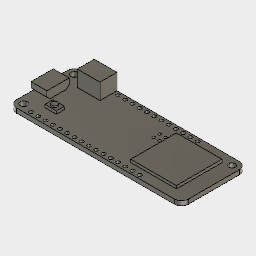
3027 Adafruit FONA Feather 32u4 (Autodesk Fusion 360 design; units mm, degrees)
Autodesk Fusion 360 part; units mm, degrees
sketch "Adafruit Feather 32u4 FONA" plane through (0, 0, 0) normal (0, 0, 1) x (1, 0, 0)
  arc A0 (1.895, 14.93) -> (2.295, 14.58) centre (2.27, 14.955) ccw
  line L0 (0, 8.89) -> (0, 2.54)
  arc A1 (60.325, 20.32) -> (57.785, 22.86) centre (57.785, 20.32) ccw
  arc A2 (2.245, 8.28) -> (1.895, 7.83) centre (2.295, 7.88) ccw
  arc A3 (57.785, 0) -> (60.325, 2.54) centre (57.785, 2.54) ccw
  line L1 (2.845, 14.58) -> (2.295, 14.58)
  line L2 (1.895, 14.93) -> (1.895, 15.13)
  arc A4 (1.895, 7.83) -> (2.245, 7.38) centre (2.295, 7.78) ccw
  arc A5 (0, 2.54) -> (2.54, 0) centre (2.54, 2.54) ccw
  arc A6 (2.845, 14.58) -> (3.195, 14.93) centre (2.845, 14.93) ccw
  arc A7 (2.54, 22.86) -> (0, 20.32) centre (2.54, 20.32) ccw
  line L3 (57.785, 22.86) -> (2.54, 22.86)
  line L4 (60.325, 2.54) -> (60.325, 20.32)
  arc A8 (2.295, 15.48) -> (1.895, 15.13) centre (2.27, 15.105) ccw
  line L5 (3.195, 15.13) -> (3.195, 14.93)
  circle A9 centre (57.785, 20.32) radius 1.1
  line L6 (2.54, 0) -> (57.785, 0)
  arc A10 (3.195, 7.83) -> (2.845, 8.28) centre (2.795, 7.88) ccw
  line L7 (0.508, 13.589) -> (0.508, 9.398)
  line L8 (2.845, 7.38) -> (2.245, 7.38)
  line L9 (0.508, 9.398) -> (0, 8.89)
  line L10 (2.245, 8.28) -> (2.845, 8.28)
  line L11 (0, 20.32) -> (0, 14.097)
  line L12 (0, 14.097) -> (0.508, 13.589)
  arc A11 (2.845, 7.38) -> (3.195, 7.83) centre (2.795, 7.78) ccw
  circle A12 centre (4.445, 13.38) radius 0.35
  arc A13 (3.195, 15.13) -> (2.845, 15.48) centre (2.845, 15.13) ccw
  circle A14 centre (4.445, 9.48) radius 0.35
  line L13 (2.295, 15.48) -> (2.845, 15.48)
  circle A15 centre (35.576, 15.113) radius 0.704
  line L14 (3.795, 9.08) -> (1.295, 9.08)
  circle A16 centre (35.576, 17.145) radius 0.704
  circle A17 centre (39.37, 1.27) radius 0.8382
  line L15 (1.295, 9.08) -> (1.295, 6.58)
  line L16 (1.295, 16.28) -> (1.295, 13.78)
  arc A18 (5.999, 8.13) -> (4.691, 8.13) centre (5.345, 8.13) ccw
  circle A19 centre (35.576, 17.145) radius 0.704
  line L17 (3.795, 16.28) -> (1.295, 16.28)
  line L18 (3.795, 6.58) -> (3.795, 9.08)
  line L19 (1.295, 9.08) -> (1.295, 6.58)
  line L20 (5.999, 6.822) -> (5.999, 8.13)
  line L21 (1.295, 13.78) -> (3.795, 13.78)
  line L22 (4.691, 8.13) -> (4.691, 6.822)
  arc A20 (5.999, 8.13) -> (4.691, 8.13) centre (5.345, 8.13) ccw
  arc A21 (4.691, 6.822) -> (5.999, 6.822) centre (5.345, 6.822) ccw
  line L23 (5.999, 6.822) -> (5.999, 8.13)
  line L24 (3.795, 13.78) -> (3.795, 16.28)
  circle A22 centre (37.576, 17.145) radius 0.704
  line L25 (3.795, 9.08) -> (1.295, 9.08)
  circle A23 centre (37.576, 17.145) radius 0.704
  line L26 (1.295, 13.78) -> (3.795, 13.78)
  arc A24 (4.691, 6.822) -> (5.999, 6.822) centre (5.345, 6.822) ccw
  line L27 (1.295, 16.28) -> (1.295, 13.78)
  line L28 (1.295, 6.58) -> (3.795, 6.58)
  arc A25 (5.999, 16.038) -> (4.691, 16.038) centre (5.345, 16.038) ccw
  line L29 (3.795, 13.78) -> (3.795, 16.28)
  line L30 (5.999, 14.73) -> (5.999, 16.038)
  line L31 (5.999, 14.73) -> (5.999, 16.038)
  arc A26 (4.691, 14.73) -> (5.999, 14.73) centre (5.345, 14.73) ccw
  arc A27 (5.999, 16.038) -> (4.691, 16.038) centre (5.345, 16.038) ccw
  line L32 (4.691, 16.038) -> (4.691, 14.73)
  line L33 (4.691, 8.13) -> (4.691, 6.822)
  line L34 (3.795, 6.58) -> (3.795, 9.08)
  arc A28 (4.691, 14.73) -> (5.999, 14.73) centre (5.345, 14.73) ccw
  line L35 (1.295, 6.58) -> (3.795, 6.58)
  line L36 (4.691, 16.038) -> (4.691, 14.73)
  circle A29 centre (37.576, 15.113) radius 0.704
  circle A30 centre (37.576, 15.113) radius 0.704
  circle A31 centre (35.576, 15.113) radius 0.704
  line L37 (3.795, 16.28) -> (1.295, 16.28)
  circle A32 centre (21.59, 21.59) radius 0.8382
  circle A33 centre (41.91, 1.27) radius 0.8382
  circle A34 centre (44.45, 1.27) radius 0.8382
  circle A35 centre (41.91, 1.27) radius 0.8382
  circle A36 centre (2.54, 20.32) radius 1.758
  circle A37 centre (2.54, 2.54) radius 1.758
  circle A38 centre (2.54, 2.54) radius 1.758
  circle A39 centre (2.54, 20.32) radius 1.758
  circle A40 centre (24.13, 21.59) radius 0.8382
  circle A41 centre (21.59, 21.59) radius 0.8382
  circle A42 centre (24.13, 21.59) radius 0.8382
  circle A43 centre (41.91, 21.59) radius 0.8382
  circle A44 centre (41.91, 21.59) radius 0.8382
  circle A45 centre (44.45, 21.59) radius 0.8382
  circle A46 centre (44.45, 21.59) radius 0.8382
  circle A47 centre (36.83, 21.59) radius 0.8382
  circle A48 centre (19.05, 21.59) radius 0.8382
  circle A49 centre (16.51, 21.59) radius 0.8382
  circle A50 centre (21.59, 1.27) radius 0.8382
  circle A51 centre (21.59, 1.27) radius 0.8382
  circle A52 centre (24.13, 1.27) radius 0.8382
  circle A53 centre (11.43, 1.27) radius 0.8382
  circle A54 centre (19.05, 21.59) radius 0.8382
  circle A55 centre (24.13, 1.27) radius 0.8382
  circle A56 centre (26.67, 1.27) radius 0.8382
  circle A57 centre (16.51, 1.27) radius 0.8382
  circle A58 centre (16.51, 1.27) radius 0.8382
  circle A59 centre (16.51, 21.59) radius 0.8382
  circle A60 centre (39.37, 21.59) radius 0.8382
  circle A61 centre (36.83, 21.59) radius 0.8382
  circle A62 centre (39.37, 21.59) radius 0.8382
  circle A63 centre (31.75, 1.27) radius 0.8382
  circle A64 centre (31.75, 1.27) radius 0.8382
  circle A65 centre (29.21, 1.27) radius 0.8382
  circle A66 centre (29.21, 1.27) radius 0.8382
  circle A67 centre (26.67, 1.27) radius 0.8382
  circle A68 centre (8.89, 1.27) radius 0.8382
  circle A69 centre (34.29, 1.27) radius 0.8382
  circle A70 centre (6.35, 1.27) radius 0.8382
  circle A71 centre (8.89, 1.27) radius 0.8382
  circle A72 centre (6.35, 1.27) radius 0.8382
  circle A73 centre (31.75, 21.59) radius 0.8382
  circle A74 centre (31.75, 21.59) radius 0.8382
  circle A75 centre (34.29, 21.59) radius 0.8382
  circle A76 centre (34.29, 1.27) radius 0.8382
  circle A77 centre (29.21, 21.59) radius 0.8382
  circle A78 centre (34.29, 21.59) radius 0.8382
  circle A79 centre (26.67, 21.59) radius 0.8382
  circle A80 centre (11.43, 1.27) radius 0.8382
  circle A81 centre (39.37, 1.27) radius 0.8382
  circle A82 centre (13.97, 1.27) radius 0.8382
  circle A83 centre (26.67, 21.59) radius 0.8382
  circle A84 centre (36.83, 1.27) radius 0.8382
  circle A85 centre (44.45, 1.27) radius 0.8382
  circle A86 centre (19.05, 1.27) radius 0.8382
  circle A87 centre (19.05, 1.27) radius 0.8382
  circle A88 centre (13.97, 1.27) radius 0.8382
  circle A89 centre (29.21, 21.59) radius 0.8382
  circle A90 centre (36.83, 1.27) radius 0.8382
  circle A91 centre (2.54, 2.54) radius 1.25
  circle A92 centre (2.54, 20.32) radius 1.25
  dimension "d1" = 2.5
  dimension "d2" = 2.5
  measures "d1" diameter of A91
  measures "d2" diameter of A92
extrude "Extrude1" add sketch "Adafruit Feather 32u4 FONA" against normal blind 1.6 contours A0 L1 L2 A6 A8 L5 A13 L13 | L0 A1 A3 A5 A7 L3 L4 L6 L7 L9 L11 L12 | A2 A4 A10 L8 L10 A11 | A12 | A14 | L14 L15 L18 L19 L25 L28 L34 L35 | L16 L17 L21 L24 L26 L27 L29 L37 | A18 L20 L22 A20 A21 L23 A24 L33 | A25 L30 L31 A26 A27 L32 A28 L36 | A36 A39 | A37 A38 makes body 1
move_face "OffsetFaces1" offset 0.203 32 faces at (44.5542, 2.1017, -1.0667) (42.0142, 2.1017, -1.0667) (39.4742, 2.1017, -1.0667) (36.9342, 2.1017, -1.0667) (34.3942, 2.1017, -1.0667) (32.2048, 1.9741, -1.0667) (30.044, 1.1865, -1.0667) (27.504, 1.1865, -1.0667) (24.964, 1.1865, -1.0667) (22.424, 1.1865, -1.0667) (19.884, 1.1865, -1.0667) (17.344, 1.1865, -1.0667) (14.804, 1.1865, -1.0667) (12.264, 1.1865, -1.0667) (9.724, 1.1865, -1.0667) (7.184, 1.1865, -1.0667) (17.3316, 21.4239, -1.0667) (19.8716, 21.4239, -1.0667) (22.4116, 21.4239, -1.0667) (24.9516, 21.4239, -1.0667) (27.4916, 21.4239, -1.0667) (30.0316, 21.4239, -1.0667) (32.2048, 22.2941, -1.0667) (33.6218, 22.0961, -1.0667) (36.1618, 22.0961, -1.0667) (38.7018, 22.0961, -1.0667) (41.2418, 22.0961, -1.0667) (43.7818, 22.0961, -1.0667) (37.958, 15.7044, -1.0667) (35.958, 15.7044, -1.0667) (35.958, 17.7364, -1.0667) (37.958, 17.7364, -1.0667) on bodies 1
sketch "microUSB" plane through (0, 0, 0) normal (0, 0, 1) x (-1, 0, 0)
  circle A0 centre (-36.83, -21.59) radius 0.6352
  circle A1 centre (-44.45, -21.59) radius 0.6352
  circle A2 centre (-29.21, -1.27) radius 0.6352
  circle A3 centre (-26.67, -1.27) radius 0.6352
  circle A4 centre (-8.89, -1.27) radius 0.6352
  circle A5 centre (-35.576, -17.145) radius 0.501
  circle A6 centre (-36.83, -1.27) radius 0.6352
  circle A7 centre (-29.21, -21.59) radius 0.6352
  circle A8 centre (-13.97, -1.27) radius 0.6352
  circle A9 centre (-19.05, -1.27) radius 0.6352
  circle A10 centre (-44.45, -1.27) radius 0.6352
  circle A11 centre (-26.67, -21.59) radius 0.6352
  circle A12 centre (-39.37, -1.27) radius 0.6352
  circle A13 centre (-39.37, -21.59) radius 0.6352
  circle A14 centre (-41.91, -1.27) radius 0.6352
  circle A15 centre (-6.35, -1.27) radius 0.6352
  circle A16 centre (-16.51, -21.59) radius 0.6352
  circle A17 centre (-16.51, -1.27) radius 0.6352
  circle A18 centre (-19.05, -21.59) radius 0.6352
  circle A19 centre (-31.75, -1.27) radius 0.6352
  circle A20 centre (-21.59, -1.27) radius 0.6352
  circle A21 centre (-11.43, -1.27) radius 0.6352
  circle A22 centre (-37.576, -15.113) radius 0.501
  circle A23 centre (-57.785, -20.32) radius 1.1
  circle A24 centre (-2.54, -20.32) radius 1.25
  circle A25 centre (-2.54, -2.54) radius 1.25
  circle A26 centre (-37.576, -17.145) radius 0.501
  circle A27 centre (-35.576, -15.113) radius 0.501
  circle A28 centre (-31.75, -21.59) radius 0.6352
  circle A29 centre (-24.13, -1.27) radius 0.6352
  circle A30 centre (-34.29, -21.59) radius 0.6352
  circle A31 centre (-41.91, -21.59) radius 0.6352
  circle A32 centre (-21.59, -21.59) radius 0.6352
  circle A33 centre (-34.29, -1.27) radius 0.6352
  circle A34 centre (-24.13, -21.59) radius 0.6352
  line L0 (0, -14.097) -> (-0.508, -13.589)
  line L1 (-0.508, -13.589) -> (-0.508, -9.398)
  line L2 (-0.508, -9.398) -> (0, -8.89)
  line L3 (0, -8.89) -> (0, -2.54)
  arc A35 (0, -2.54) -> (-2.54, 0) centre (-2.54, -2.54) ccw
  line L4 (-2.54, 0) -> (-57.785, 0)
  arc A36 (-57.785, 0) -> (-60.325, -2.54) centre (-57.785, -2.54) ccw
  line L5 (-60.325, -2.54) -> (-60.325, -20.32)
  arc A37 (-60.325, -20.32) -> (-57.785, -22.86) centre (-57.785, -20.32) ccw
  line L6 (-57.785, -22.86) -> (-2.54, -22.86)
  arc A38 (-2.54, -22.86) -> (0, -20.32) centre (-2.54, -20.32) ccw
  line L7 (0, -20.32) -> (0, -14.097)
  line L8 (-0.508, -11.4935) -> (-60.325, -11.43) construction
  line L9 (0, -15.391) -> (-5.6, -15.391)
  line L10 (-5.6, -15.391) -> (-5.6, -7.591)
  line L11 (-5.6, -7.591) -> (0, -7.591)
  line L12 (0, -7.591) -> (0, -15.391)
  line L13 (-5.6, -11.491) -> (0, -11.491) construction
  line L14 (0, -14.097) -> (0, -8.89) construction
  dimension "d9" = 11.369
  dimension "d10" = 7.8
  dimension "d11" = 5.6
  measures "d9" distance of L6 L13
  measures "d10" distance of L9.end L10.end
  measures "d11" distance of L9.start L9.end
extrude "Extrude2" add sketch "microUSB" along normal blind 2.95 separate body contours L0 L1 L2 L3 L7 L9 L10 L11 L12 | L0 L1 L2 L12 makes body 2
chamfer "Chamfer1" distance 1 angle 45 2 edges at (2.8, 7.591, 0) (2.8, 15.391, 0) on bodies 2
sketch "JST 2-pin" plane through (0, 0, 0) normal (0, 0, 1) x (-1, 0, 0)
  circle A0 centre (-36.83, -21.59) radius 0.6352
  circle A1 centre (-44.45, -21.59) radius 0.6352
  circle A2 centre (-29.21, -1.27) radius 0.6352
  circle A3 centre (-26.67, -1.27) radius 0.6352
  circle A4 centre (-8.89, -1.27) radius 0.6352
  circle A5 centre (-35.576, -17.145) radius 0.501
  circle A6 centre (-36.83, -1.27) radius 0.6352
  circle A7 centre (-29.21, -21.59) radius 0.6352
  circle A8 centre (-13.97, -1.27) radius 0.6352
  circle A9 centre (-19.05, -1.27) radius 0.6352
  circle A10 centre (-44.45, -1.27) radius 0.6352
  circle A11 centre (-26.67, -21.59) radius 0.6352
  circle A12 centre (-39.37, -1.27) radius 0.6352
  circle A13 centre (-39.37, -21.59) radius 0.6352
  circle A14 centre (-41.91, -1.27) radius 0.6352
  circle A15 centre (-6.35, -1.27) radius 0.6352
  circle A16 centre (-16.51, -21.59) radius 0.6352
  circle A17 centre (-16.51, -1.27) radius 0.6352
  circle A18 centre (-19.05, -21.59) radius 0.6352
  circle A19 centre (-31.75, -1.27) radius 0.6352
  circle A20 centre (-21.59, -1.27) radius 0.6352
  circle A21 centre (-11.43, -1.27) radius 0.6352
  circle A22 centre (-37.576, -15.113) radius 0.501
  circle A23 centre (-57.785, -20.32) radius 1.1
  circle A24 centre (-2.54, -20.32) radius 1.25
  circle A25 centre (-2.54, -2.54) radius 1.25
  circle A26 centre (-37.576, -17.145) radius 0.501
  circle A27 centre (-35.576, -15.113) radius 0.501
  circle A28 centre (-31.75, -21.59) radius 0.6352
  circle A29 centre (-24.13, -1.27) radius 0.6352
  circle A30 centre (-34.29, -21.59) radius 0.6352
  circle A31 centre (-41.91, -21.59) radius 0.6352
  circle A32 centre (-21.59, -21.59) radius 0.6352
  circle A33 centre (-34.29, -1.27) radius 0.6352
  circle A34 centre (-24.13, -21.59) radius 0.6352
  line L0 (0, -14.097) -> (-0.508, -13.589)
  line L1 (-0.508, -13.589) -> (-0.508, -9.398)
  line L2 (-0.508, -9.398) -> (0, -8.89)
  line L3 (0, -8.89) -> (0, -2.54)
  arc A35 (0, -2.54) -> (-2.54, 0) centre (-2.54, -2.54) ccw
  line L4 (-2.54, 0) -> (-57.785, 0)
  arc A36 (-57.785, 0) -> (-60.325, -2.54) centre (-57.785, -2.54) ccw
  line L5 (-60.325, -2.54) -> (-60.325, -20.32)
  arc A37 (-60.325, -20.32) -> (-57.785, -22.86) centre (-57.785, -20.32) ccw
  line L6 (-57.785, -22.86) -> (-2.54, -22.86)
  arc A38 (-2.54, -22.86) -> (0, -20.32) centre (-2.54, -20.32) ccw
  line L7 (0, -20.32) -> (0, -14.097)
  line L8 (-6.92, -22.86) -> (-14.92, -22.86)
  line L9 (-14.92, -22.86) -> (-14.92, -16.86)
  line L10 (-14.92, -16.86) -> (-6.92, -16.86)
  line L11 (-6.92, -16.86) -> (-6.92, -22.86)
  line L12 (-10.92, -22.86) -> (-10.92, -16.86) construction
  dimension "d15" = 8
  dimension "d16" = 6
  dimension "d17" = 10.92
  measures "d15" distance of L8.start L8.end
  measures "d16" distance of L8.end L9.end
  measures "d17" distance of L7 L12
extrude "Extrude3" add sketch "JST 2-pin" along normal blind 5.6 separate body contours L6 L8 L9 L10 L11 makes body 3
sketch "sim800h" plane through (0, 0, 0) normal (0, 0, 1) x (-1, 0, 0)
  circle A0 centre (-36.83, -21.59) radius 0.6352
  circle A1 centre (-44.45, -21.59) radius 0.6352
  circle A2 centre (-29.21, -1.27) radius 0.6352
  circle A3 centre (-26.67, -1.27) radius 0.6352
  circle A4 centre (-8.89, -1.27) radius 0.6352
  circle A5 centre (-35.576, -17.145) radius 0.501
  circle A6 centre (-36.83, -1.27) radius 0.6352
  circle A7 centre (-29.21, -21.59) radius 0.6352
  circle A8 centre (-13.97, -1.27) radius 0.6352
  circle A9 centre (-19.05, -1.27) radius 0.6352
  circle A10 centre (-44.45, -1.27) radius 0.6352
  circle A11 centre (-26.67, -21.59) radius 0.6352
  circle A12 centre (-39.37, -1.27) radius 0.6352
  circle A13 centre (-39.37, -21.59) radius 0.6352
  circle A14 centre (-41.91, -1.27) radius 0.6352
  circle A15 centre (-6.35, -1.27) radius 0.6352
  circle A16 centre (-16.51, -21.59) radius 0.6352
  circle A17 centre (-16.51, -1.27) radius 0.6352
  circle A18 centre (-19.05, -21.59) radius 0.6352
  circle A19 centre (-31.75, -1.27) radius 0.6352
  circle A20 centre (-21.59, -1.27) radius 0.6352
  circle A21 centre (-11.43, -1.27) radius 0.6352
  circle A22 centre (-37.576, -15.113) radius 0.501
  circle A23 centre (-57.785, -20.32) radius 1.1
  circle A24 centre (-2.54, -20.32) radius 1.25
  circle A25 centre (-2.54, -2.54) radius 1.25
  circle A26 centre (-37.576, -17.145) radius 0.501
  circle A27 centre (-35.576, -15.113) radius 0.501
  circle A28 centre (-31.75, -21.59) radius 0.6352
  circle A29 centre (-24.13, -1.27) radius 0.6352
  circle A30 centre (-34.29, -21.59) radius 0.6352
  circle A31 centre (-41.91, -21.59) radius 0.6352
  circle A32 centre (-21.59, -21.59) radius 0.6352
  circle A33 centre (-34.29, -1.27) radius 0.6352
  circle A34 centre (-24.13, -21.59) radius 0.6352
  line L0 (0, -14.097) -> (-0.508, -13.589)
  line L1 (-0.508, -13.589) -> (-0.508, -9.398)
  line L2 (-0.508, -9.398) -> (0, -8.89)
  line L3 (0, -8.89) -> (0, -2.54)
  arc A35 (0, -2.54) -> (-2.54, 0) centre (-2.54, -2.54) ccw
  line L4 (-2.54, 0) -> (-57.785, 0)
  arc A36 (-57.785, 0) -> (-60.325, -2.54) centre (-57.785, -2.54) ccw
  line L5 (-60.325, -2.54) -> (-60.325, -20.32)
  arc A37 (-60.325, -20.32) -> (-57.785, -22.86) centre (-57.785, -20.32) ccw
  line L6 (-57.785, -22.86) -> (-2.54, -22.86)
  arc A38 (-2.54, -22.86) -> (0, -20.32) centre (-2.54, -20.32) ccw
  line L7 (0, -20.32) -> (0, -14.097)
  line L8 (-55.117, -3.43) -> (-39.117, -3.43)
  line L9 (-39.117, -3.43) -> (-39.117, -19.43)
  line L10 (-39.117, -19.43) -> (-55.117, -19.43)
  line L11 (-55.117, -19.43) -> (-55.117, -3.43)
  line L12 (-55.117, -3.43) -> (-39.117, -19.43) construction
  line L13 (-39.117, -3.43) -> (-55.117, -19.43) construction
  point P0 (-47.117, -11.43)
  dimension "d20" = 16
  dimension "d21" = 16
  dimension "d22" = 11.43
  dimension "d23" = 47.117
  measures "d20" distance of L8.end L9.end
  measures "d21" distance of L9.end L10.end
  measures "d22" distance of L4 P0
  measures "d23" distance of L3 P0
extrude "Extrude4" add sketch "sim800h" along normal blind 1 separate body contours L8 L9 L10 L11 makes body 4
sketch "reset switch" plane through (0, 0, 0) normal (0, 0, 1) x (-1, 0, 0)
  circle A0 centre (-36.83, -21.59) radius 0.6352
  circle A1 centre (-44.45, -21.59) radius 0.6352
  circle A2 centre (-29.21, -1.27) radius 0.6352
  circle A3 centre (-26.67, -1.27) radius 0.6352
  circle A4 centre (-8.89, -1.27) radius 0.6352
  circle A5 centre (-35.576, -17.145) radius 0.501
  circle A6 centre (-36.83, -1.27) radius 0.6352
  circle A7 centre (-29.21, -21.59) radius 0.6352
  circle A8 centre (-13.97, -1.27) radius 0.6352
  circle A9 centre (-19.05, -1.27) radius 0.6352
  circle A10 centre (-44.45, -1.27) radius 0.6352
  circle A11 centre (-26.67, -21.59) radius 0.6352
  circle A12 centre (-39.37, -1.27) radius 0.6352
  circle A13 centre (-39.37, -21.59) radius 0.6352
  circle A14 centre (-41.91, -1.27) radius 0.6352
  circle A15 centre (-6.35, -1.27) radius 0.6352
  circle A16 centre (-16.51, -21.59) radius 0.6352
  circle A17 centre (-16.51, -1.27) radius 0.6352
  circle A18 centre (-19.05, -21.59) radius 0.6352
  circle A19 centre (-31.75, -1.27) radius 0.6352
  circle A20 centre (-21.59, -1.27) radius 0.6352
  circle A21 centre (-11.43, -1.27) radius 0.6352
  circle A22 centre (-37.576, -15.113) radius 0.501
  circle A23 centre (-57.785, -20.32) radius 1.1
  circle A24 centre (-2.54, -20.32) radius 1.25
  circle A25 centre (-2.54, -2.54) radius 1.25
  circle A26 centre (-37.576, -17.145) radius 0.501
  circle A27 centre (-35.576, -15.113) radius 0.501
  circle A28 centre (-31.75, -21.59) radius 0.6352
  circle A29 centre (-24.13, -1.27) radius 0.6352
  circle A30 centre (-34.29, -21.59) radius 0.6352
  circle A31 centre (-41.91, -21.59) radius 0.6352
  circle A32 centre (-21.59, -21.59) radius 0.6352
  circle A33 centre (-34.29, -1.27) radius 0.6352
  circle A34 centre (-24.13, -21.59) radius 0.6352
  line L0 (0, -14.097) -> (-0.508, -13.589)
  line L1 (-0.508, -13.589) -> (-0.508, -9.398)
  line L2 (-0.508, -9.398) -> (0, -8.89)
  line L3 (0, -8.89) -> (0, -2.54)
  arc A35 (0, -2.54) -> (-2.54, 0) centre (-2.54, -2.54) ccw
  line L4 (-2.54, 0) -> (-57.785, 0)
  arc A36 (-57.785, 0) -> (-60.325, -2.54) centre (-57.785, -2.54) ccw
  line L5 (-60.325, -2.54) -> (-60.325, -20.32)
  arc A37 (-60.325, -20.32) -> (-57.785, -22.86) centre (-57.785, -20.32) ccw
  line L6 (-57.785, -22.86) -> (-2.54, -22.86)
  arc A38 (-2.54, -22.86) -> (0, -20.32) centre (-2.54, -20.32) ccw
  line L7 (0, -20.32) -> (0, -14.097)
  line L8 (-11.398, -5.077) -> (-7.398, -5.077)
  line L9 (-7.398, -5.077) -> (-7.398, -7.877)
  line L10 (-7.398, -7.877) -> (-11.398, -7.877)
  line L11 (-11.398, -7.877) -> (-11.398, -5.077)
  line L12 (-11.398, -5.077) -> (-7.398, -7.877) construction
  line L13 (-7.398, -5.077) -> (-11.398, -7.877) construction
  circle A39 centre (-9.398, -6.477) radius 1
  point P0 (-9.398, -6.477)
  dimension "d26" = 4
  dimension "d27" = 2.8
  dimension "d28" = 9.398
  dimension "d29" = 6.477
  dimension "d30" = 2
  measures "d26" distance of L9.end L10.end
  measures "d27" distance of L8.end L9.end
  measures "d28" distance of L3 P0
  measures "d29" distance of L4 P0
  measures "d30" diameter of A39
extrude "Extrude5" add sketch "reset switch" along normal blind 1 separate body contours L8 L9 L10 L11 | A39 makes body 5
extrude "Extrude6" add sketch "reset switch" along normal blind 0.5 from surface at 1 contours A39 bodies 5
equation "d6 = ( 0.406 / 2 ) * 1 mm"
named bodies: "pcb", "microUSB", "jst", "sim800h", "reset switch"
